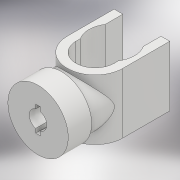
# Autodesk Inventor part: Laser Mount
Saved by Autodesk Inventor 2018.2 (Build 222227000, 227)
## iProperties
Created: 2018-01-13
Part Number: Laser Mount
Material: ABS Plastic
Document SubType Name: Modeling
Designer: Moochster
Density: 1.06 g/cm^3
Appearance: Smooth - White
Mass: 0.636628 g
Surface Area: 8.23061 cm^2
Volume: 0.600592 cm^3
Author: Moochster
Autodesk Inventor part; units mm, degrees
ref_plane "YZ Plane" through (0, 0, 0) normal (1, 0, 0) x (0, 1, 0)
ref_plane "XZ Plane" through (0, 0, 0) normal (0, 1, 0) x (-1, 0, 0)
ref_plane "XY Plane" through (0, 0, 0) normal (0, 0, 1) x (1, 0, 0)
sketch "Sketch1" plane through (0, 0, 0) normal (0, 1, 0) x (-1, 0, 0)
  circle A0 centre (0, 0) radius 1.05 construction
  arc A1 (-0.35, 1.2624) -> (-0.35, -1.2624) centre (0, 0) ccw
  circle A2 centre (0, 0) radius 4.5
  line L0 (0.35, 1.875) -> (-0.35, 1.875)
  line L1 (-0.35, 1.875) -> (-0.35, -1.875)
  line L2 (-0.35, -1.875) -> (0.35, -1.875)
  line L3 (0.35, -1.875) -> (0.35, 1.875)
  arc A3 (0.35, 1.2624) -> (-0.35, 1.2624) centre (0, 0) ccw
  arc A4 (0.35, -1.2624) -> (0.35, 1.2624) centre (0, 0) ccw
  arc A5 (-0.35, -1.2624) -> (0.35, -1.2624) centre (0, 0) ccw
  point P0 (0, 1.875)
  point P1 (0.35, 0)
  dimension "d1" = 2.1
  dimension "d3" = 9
  dimension "d18" = 0.26
  dimension "d19" = 0.7
  dimension "d20" = 3.75
  constraints: 8 end point, 8 point on circle, 6 centre point, 4 point on line, 3 coincident, 2 midpoint, 2 parallel, 1 horizontal, 1 horizontal alignment, 1 perpendicular, 1 vertical alignment
  measures "d1" diameter of A0
  measures "d3" diameter of A2
  measures "d18" radial gap between concentric circles of A1 A0
  measures "d19" distance of L0.start L0.end
  measures "d20" distance of L0.end L1.end
extrude "Extrusion1" add sketch "Sketch1" along normal blind 3.5
sketch "Sketch4" plane through (0, 0, 0) normal (0, 0, 1) x (1, 0, 0)
  line L0 (-4.15, 15.5) -> (-4.15, 8.5)
  arc A0 (-4.15, 8.5) -> (4.15, 8.5) centre (0, 8.5) ccw
  line L1 (4.15, 8.5) -> (4.15, 15.5)
  line L2 (-2.85, 15.5) -> (-2.85, 12.854)
  arc A1 (-2.85, 8.5) -> (2.85, 8.5) centre (0, 8.5) ccw
  line L3 (2.85, 8.5) -> (2.85, 9.146)
  line L4 (-4.15, 15.5) -> (-2.85, 15.5)
  line L5 (2.85, 15.5) -> (4.15, 15.5)
  line L6 (-0.35, 0) -> (0.35, 0) projected
  line L7 (4.5, 3.5) -> (-4.5, 3.5) projected
  circle A2 centre (0, 11) radius 3.4
  line L8 (-2.85, 12.854) -> (-2.85, 9.146)
  line L9 (-2.85, 9.146) -> (-2.85, 8.5)
  line L10 (2.85, 9.146) -> (2.85, 12.854)
  line L11 (2.85, 12.854) -> (2.85, 15.5)
  point P0 (0, 0)
  point P1 (0, 0)
  dimension "d21" = 2.85
  dimension "d23" = 1.3
  dimension "d24" = 5
  dimension "d25" = 7
  dimension "d26" = 6.8
  dimension "d27" = 2.5
  constraints: 20 end point, 10 parallel, 8 point on circle, 4 tangent, 3 centre point, 2 vertical, 2 vertical alignment, 1 collinear, 1 horizontal, 1 horizontal alignment, 1 midpoint
  measures "d21" radius of A1
  measures "d23" distance of L5.start L1.end
  measures "d24" distance from line of L7 A0.centre
  measures "d25" distance of L1.start L1.end
  measures "d26" diameter of A2
  measures "d27" distance of A0.centre A2.centre
extrude "Extrusion5" add sketch "Sketch4" along normal mid plane 9 contours L4 L2 A2 L9 A1 L3 L11 L5 L1 A0 L0
sketch "Sketch8" plane through (0, 3.5, 0) normal (0, 1, 0) x (1, 0, 0)
  circle A0 centre (0, 0) radius 4
  arc A1 (0.35, -1.2624) -> (0.35, 1.2624) centre (0, 0) ccw projected
  line L0 (0.35, 1.875) -> (0.35, 1.2624) projected
  line L1 (-0.35, 1.875) -> (0.35, 1.875) projected
  line L2 (-0.35, 1.2624) -> (-0.35, 1.875) projected
  arc A2 (-0.35, 1.2624) -> (-0.35, -1.2624) centre (0, 0) ccw projected
  line L3 (-0.35, -1.875) -> (-0.35, -1.2624) projected
  line L4 (0.35, -1.875) -> (-0.35, -1.875) projected
  line L5 (0.35, -1.2624) -> (0.35, -1.875) projected
  dimension "d33" = 8
  constraints: 1 centre point, 1 coincident
  measures "d33" diameter of A0
extrude "Extrusion6" add sketch "Sketch8" along normal up to next
sketch "Sketch2" plane through (0, 3.5, 0) normal (0, 1, 0) x (1, 0, 0)
  circle A0 centre (0, 0) radius 1.31 projected
  circle A1 centre (0, 0) radius 3.31
  dimension "d6" = 2
  dimension "d9" = 7.3
  dimension "d10" = 2
  constraints: 6 end point, 4 point on circle, 3 midpoint, 2 centre point, 2 line through centre, 1 coincident, 1 horizontal, 1 perpendicular, 1 vertical alignment
body "Solid1"
